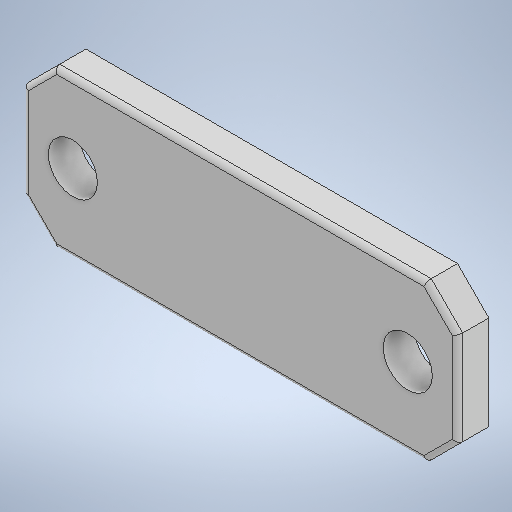
# Autodesk Inventor part: MagneticLimitBaseSpacer3milTall
Saved by Autodesk Inventor 2025.2 (Build 292293000, 293)
## iProperties
Created: 2025-02-28
Part Number: MagneticLimitBaseSpacer3milTall
Material: Generic
Document SubType Name: Modeling
Designer: cutterj
Density: 1 g/cm^3
Appearance: Default
Author: cutterj
Autodesk Inventor part; units mm, degrees
ref_plane "YZ Plane" through (0, 0, 0) normal (1, 0, 0) x (0, 1, 0)
ref_plane "XZ Plane" through (0, 0, 0) normal (0, 1, 0) x (-1, 0, 0)
ref_plane "XY Plane" through (0, 0, 0) normal (0, 0, 1) x (1, 0, 0)
sketch "Sketch1" plane through (0, 0, 0) normal (0, 0, 1) x (1, 0, 0)
  line L0 (0, 0) -> (41.5, 0)
  line L1 (41.5, 0) -> (41.5, 15)
  line L2 (41.5, 15) -> (0, 15)
  line L3 (0, 15) -> (0, 0)
  line L4 (0, 7.5) -> (41.5, 7.5) construction
  line L5 (20.75, 15) -> (20.75, 0) construction
  circle A0 centre (20.75, 7.5) radius 16 construction
  circle A1 centre (4.75, 7.5) radius 2.35
  circle A2 centre (36.75, 7.5) radius 2.35
  dimension "d0" = 41.5
  dimension "d1" = 15
  dimension "d2" = 32
  dimension "d3" = 4.7
  dimension "d4" = 4.7
  constraints: 12 end point, 5 midpoint, 3 centre point, 2 parallel, 2 point on circle, 2 point on line, 1 horizontal, 1 perpendicular
  measures "d0" distance of L2.end L1.end
  measures "d1" distance of L1.end L0.end
  measures "d2" diameter of A0
  measures "d3" diameter of A1
  measures "d4" diameter of A2
extrude "Extrusion1" add sketch "Sketch1" along normal blind 3
chamfer "Chamfer1" distance 3 angle 45 4 edges at (0, 15, 1.5) (41.5, 15, 1.5) (41.5, 0, 1.5) (0, 0, 1.5)
fillet "Fillet1" radius 0.5 8 edges at (1.5, 1.5, 3) (20.75, 0, 3) (40, 1.5, 3) (41.5, 7.5, 3) (40, 13.5, 3) (20.75, 15, 3) (1.5, 13.5, 3) (0, 7.5, 3)
body "Solid1"
